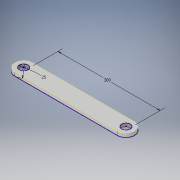
# Autodesk Inventor part: test
Saved by Autodesk Inventor 2019 (Build 230136000, 136)
## iProperties
Created: 2021-02-06
Part Number: test
Material: 一般
Document SubType Name: Modeling
Designer: wasd5
Density: 1 g/cm^3
Appearance: 預設
Author: wasd5
Autodesk Inventor part; units mm, degrees
ref_plane "YZ Plane" through (0, 0, 0) normal (1, 0, 0) x (0, 1, 0)
ref_plane "XZ Plane" through (0, 0, 0) normal (0, 1, 0) x (-1, 0, 0)
ref_plane "XY Plane" through (0, 0, 0) normal (0, 0, 1) x (1, 0, 0)
sketch "草圖1" plane through (0, 0, 0) normal (0, 1, 0) x (-1, 0, 0)
  arc A0 (0, -25) -> (0, 25) centre (0, 0) ccw
  line L0 (0, -25) -> (-300, -25)
  line L1 (-300, -25) -> (-300, 25) construction
  line L2 (-300, 25) -> (0, 25)
  line L3 (0, 25) -> (0, -25) construction
  arc A1 (-300, 25) -> (-300, -25) centre (-300, 0) ccw
  dimension "diameter" = 50
  dimension "center_length" = 300
  constraints: 8 end point, 4 point on circle, 2 centre point, 2 parallel, 2 tangent, 1 coincident, 1 horizontal, 1 midpoint, 1 perpendicular
  measures "diameter" diameter of A0
  measures "center_length" distance of L0.start L0.end
extrude "thickness" add sketch "草圖1" along normal blind 10
sketch "草圖2" plane through (0, 10, 0) normal (0, 1, 0) x (1, 0, 0)
  circle A0 centre (0, 0) radius 12.5
  arc A1 (0, 25) -> (0, -25) centre (0, 0) ccw construction
  line L0 (0, -25) -> (300, -25) construction
  arc A2 (300, -25) -> (300, 25) centre (300, 0) ccw construction
  line L1 (300, 25) -> (0, 25) construction
  circle A3 centre (300, 0) radius 12.5
  dimension "hole" = 25
  constraints: 2 centre point, 2 coincident, 1 equal radius
  measures "hole" diameter of A0
extrude "擠出2" cut sketch "草圖2" against normal up to surface (10 mm away)
